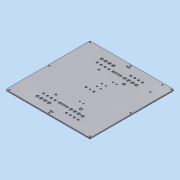
# Autodesk Inventor part: V-Slot Universal Build Pate
Saved by Autodesk Inventor 2013 (Build 170138000, 138)
## iProperties
Created: 2013-12-08
Part Number: V-Slot Universal Build Pate
Material: Aluminum 6061
Document SubType Name: Modeling
Designer: Jon Hollander
Density: 2.71 g/cm^3
Catalog Web Link: www.openbuildspartstore.com
Vendor: OpenBuilds
Mass: 366.388 g
Surface Area: 959.613 cm^2
Volume: 135.198 cm^3
Author: Work
Autodesk Inventor part; units mm, degrees
ref_plane "YZ Plane" through (0, 0, 0) normal (1, 0, 0) x (0, 1, 0)
ref_plane "XZ Plane" through (0, 0, 0) normal (0, 1, 0) x (-1, 0, 0)
ref_plane "XY Plane" through (0, 0, 0) normal (0, 0, 1) x (1, 0, 0)
sketch "Sketch1" plane through (0, 0, 0) normal (0, 0, 1) x (1, 0, 0)
  line L0 (-108, 108) -> (108, 108)
  line L1 (108, 108) -> (108, -108)
  line L2 (108, -108) -> (-108, -108)
  line L3 (-108, -108) -> (-108, 108)
  line L4 (-108, 108) -> (108, -108) construction
  line L5 (108, 108) -> (-108, -108) construction
  point P0 (0, 0)
  dimension "d0" = 216
  dimension "d2" = 216
  constraints: 12 end point, 2 midpoint, 2 parallel, 1 horizontal, 1 perpendicular
  measures "d0" distance of L1.end L2.end
  measures "d2" distance of L2.end L0.start
extrude "Extrusion1" add sketch "Sketch1" along normal mid plane 3
sketch "Sketch2" plane through (0, 0, 1.5) normal (0, 0, 1) x (1, 0, 0)
  line L0 (108, 108) -> (-108, 108) projected
  line L1 (-108, 108) -> (-108, -108) projected
  line L2 (-108, -108) -> (108, -108) projected
  line L3 (108, -108) -> (108, 108) projected
  circle A0 centre (104.5, -104.5) radius 1.8 construction
  line L4 (102.7, -104.5) -> (-104.5, -104.5) construction
  line L5 (104.5, 104.5) -> (-104.5, 104.5) construction
  line L6 (104.5, 104.5) -> (104.5, -104.5) construction
  line L7 (-104.5, 104.5) -> (-104.5, -104.5) construction
  line L8 (0, 104.5) -> (0, -104.5) construction
  point P0 (0, 0)
  point P1 (-102.3056, -104.5)
  point P2 (104.5, 0)
  point P3 (-104.5, 0)
  point P4 (0, 0)
  dimension "d6" = 3.6
  dimension "d5" = 3.5
  dimension "d7" = 1.7
  dimension "d8" = 3.5
  dimension "d9" = 3.5
  dimension "d10" = 3.5
  dimension "d11" = 3.5
  dimension "d13" = 108
  constraints: 10 end point, 3 coincident, 3 midpoint, 3 perpendicular, 2 point on line, 1 horizontal alignment, 1 parallel, 2 other
  measures "d5" distance from line of L3 point (104.5, -104.5)
  measures "d8" distance between parallel lines of L2 L4
  measures "d9" distance between parallel lines of L0 L5
  measures "d10" distance from line of L3 point (104.5, 104.5)
  measures "d11" distance between parallel lines of L1 L7
  measures "d13" distance from line of L3 L8.start
hole "Hole1" at (104.5, 104.5, 1.5) at (104.5, -104.5, 1.5) at (-102.3056, -104.5, 1.5) at (-104.5, 104.5, 1.5) at (104.5, 0, 1.5) at (-104.5, 0, 1.5) at (0, 104.5, 1.5) at (0, -104.5, 1.5) at (0, 0, 1.5) direction (0, 0, -1) diameter 3.6 end through all
sketch "Sketch3" plane through (0, 0, 1.5) normal (0, 0, 1) x (1, 0, 0)
  line L0 (108, 108) -> (-108, 108) projected
  line L1 (-108, 108) -> (-108, -108) projected
  line L2 (108, -108) -> (108, 108) projected
  line L3 (-108, 82.65) -> (108, 82.65) construction
  line L4 (-108, 69) -> (108, 69) construction
  point P0 (-52.3, 82.65)
  point P1 (-42.3, 82.65)
  point P2 (-32.3, 82.65)
  point P3 (-22.3, 82.65)
  point P4 (20.32, 69)
  point P5 (30.32, 69)
  point P6 (40.32, 69)
  point P7 (50.32, 69)
  dimension "d21" = 25.35
  dimension "d23" = 39
  dimension "d24" = 160.3
  dimension "d25" = 150.3
  dimension "d26" = 140.3
  dimension "d27" = 130.3
  dimension "d28" = 57.68
  dimension "d29" = 67.68
  dimension "d30" = 77.68
  dimension "d31" = 87.68
  constraints: 12 point on line, 4 end point, 2 perpendicular
  measures "d21" distance between parallel lines of L0 L3
  measures "d23" distance between parallel lines of L0 L4
  measures "d24" distance from line of L2 point (-52.3, 82.65)
  measures "d25" horizontal distance of L4.end point (-42.3, 82.65)
  measures "d26" distance from line of L2 point (-32.3, 82.65)
  measures "d27" distance from line of L2 point (-22.3, 82.65)
  measures "d28" distance from line of L2 point (50.32, 69)
  measures "d29" distance from line of L2 point (40.32, 69)
  measures "d30" distance from line of L2 point (30.32, 69)
  measures "d31" distance from line of L2 point (20.32, 69)
hole "Hole2" at (-52.3, 82.65, 1.5) at (-42.3, 82.65, 1.5) at (-32.3, 82.65, 1.5) at (-22.3, 82.65, 1.5) at (20.32, 69, 1.5) at (30.32, 69, 1.5) at (40.32, 69, 1.5) at (50.32, 69, 1.5) direction (0, 0, -1) diameter 7.14 end through all
sketch "Sketch4" plane through (0, 0, 1.5) normal (0, 0, 1) x (1, 0, 0)
  line L0 (-108, 108) -> (-108, -108) projected
  line L1 (108, -108) -> (108, 108) projected
  line L2 (-108, 82.65) -> (108, 82.65) construction
  line L3 (-108, 69) -> (108, 69) construction
  point P0 (-50.32, 69)
  point P1 (-40.32, 69)
  point P2 (-30.32, 69)
  point P3 (-20.32, 69)
  point P4 (22.3, 82.65)
  point P5 (32.3, 82.65)
  point P6 (42.3, 82.65)
  point P7 (52.3, 82.65)
  dimension "d125" = 158.32
  dimension "d126" = 148.32
  dimension "d127" = 138.32
  dimension "d128" = 128.32
  dimension "d129" = 55.7
  dimension "d130" = 65.7
  dimension "d131" = 75.7
  dimension "d132" = 85.7
  constraints: 12 point on line, 4 end point, 2 perpendicular
  measures "d125" distance from line of L1 point (-50.32, 69)
  measures "d126" distance from line of L1 point (-40.32, 69)
  measures "d127" distance from line of L1 point (-30.32, 69)
  measures "d128" distance from line of L1 point (-20.32, 69)
  measures "d129" distance from line of L1 point (52.3, 82.65)
  measures "d130" distance from line of L1 point (42.3, 82.65)
  measures "d131" distance from line of L1 point (32.3, 82.65)
  measures "d132" distance from line of L1 point (22.3, 82.65)
hole "Hole3" at (-50.32, 69, 1.5) at (-40.32, 69, 1.5) at (-30.32, 69, 1.5) at (-20.32, 69, 1.5) at (22.3, 82.65, 1.5) at (32.3, 82.65, 1.5) at (42.3, 82.65, 1.5) at (52.3, 82.65, 1.5) direction (0, 0, -1) diameter 5 end through all
sketch "Sketch5" plane through (0, 0, 1.5) normal (0, 0, 1) x (1, 0, 0)
  circle A0 centre (0, 0) radius 1.8 projected
  line L0 (-108, 108) -> (-108, -108) projected
  line L1 (108, -108) -> (108, 108) projected
  line L2 (-108, 55.35) -> (108, 55.35) construction
  point P0 (-32.3, 55.35)
  dimension "d46" = 55.35
  dimension "d47" = 75.7
  constraints: 3 point on line, 2 end point, 1 perpendicular
  measures "d46" distance from line of A0.centre L2
  measures "d47" distance from line of L0 point (-32.3, 55.35)
hole "Hole4" at (-32.3, 55.35, 1.5) direction (0, 0, -1) diameter 5 end through all
sketch "Sketch6" plane through (0, 0, 1.5) normal (0, 0, 1) x (1, 0, 0)
  circle A0 centre (-32.3, 55.35) radius 2.5 projected
  point P0 (32.3, 55.35)
  dimension "d55" = 64.6
  constraints: 1 horizontal alignment
  measures "d55" distance of A0.centre point (32.3, 55.35)
hole "Hole5" at (32.3, 55.35, 1.5) direction (0, 0, -1) diameter 7.14 end through all
mirror "Mirror1" about plane through (0, 0, 0) normal (0, 1, 0) of "Hole2", "Hole3", "Hole4", "Hole5"
sketch "Sketch7" plane through (0, 0, 1.5) normal (0, 0, 1) x (1, 0, 0)
  circle A0 centre (0, 0) radius 1.8 projected
  point P0 (-10, 0)
  point P1 (10, 0)
  dimension "d63" = 10
  dimension "d64" = 10
  measures "d63" distance of A0.centre point (-10, 0)
  measures "d64" distance of A0.centre point (10, 0)
hole "Hole6" at (-10, 0, 1.5) at (10, 0, 1.5) direction (0, 0, -1) diameter 5 end through all
sketch "Sketch8" plane through (0, 0, 1.5) normal (0, 0, 1) x (1, 0, 0)
  line L0 (108, 108) -> (-108, 108) projected
  line L1 (-108, 108) -> (-108, -108) projected
  line L2 (108, -108) -> (108, 108) projected
  line L3 (2.5, 15.2915) -> (2.5, 28) construction
  point P0 (12.64, 15.17)
  point P1 (12.64, 28)
  dimension "d72" = 80
  dimension "d73" = 10.14
  dimension "d74" = 12.83
  dimension "d75" = 110.5
  constraints: 2 end point, 2 parallel, 1 coincident, 1 horizontal alignment, 1 vertical alignment
  measures "d72" distance from line of L0 point (12.64, 28)
  measures "d73" distance of L3.end point (12.64, 28)
  measures "d74" distance of point (12.64, 28) point (12.64, 15.17)
  measures "d75" distance from line of L1 point (2.5, 15.291)
hole "Hole7" at (2.5, 15.2915, 1.5) at (12.64, 15.17, 1.5) at (12.64, 28, 1.5) at (2.5, 28, 1.5) direction (0, 0, -1) diameter 3.5 end through all
sketch "Sketch9" plane through (0, 0, 1.5) normal (0, 0, 1) x (1, 0, 0)
  line L0 (108, 108) -> (-108, 108) projected
  line L1 (-108, 108) -> (-108, -108) projected
  point P0 (14, 45)
  point P1 (23.12, 45)
  dimension "d83" = 122
  dimension "d84" = 63
  dimension "d85" = 9.12
  measures "d83" distance from line of L1 point (14, 45)
  measures "d84" distance from line of L0 point (14, 45)
  measures "d85" distance of point (23.12, 45) point (14, 45)
hole "Hole8" at (14, 45, 1.5) at (23.12, 45, 1.5) direction (0, 0, -1) diameter 3.14 end through all
sketch "Sketch10" plane through (0, 0, 1.5) normal (0, 0, 1) x (1, 0, 0)
  circle A0 centre (14, 45) radius 1.57 projected
  line L0 (-108, -108) -> (108, -108) projected
  line L1 (108, -108) -> (108, 108) projected
  line L2 (14, 45) -> (14, -40) construction
  point P0 (23.12, -40)
  dimension "d93" = 68
  dimension "d94" = 9.12
  constraints: 2 end point, 1 coincident, 1 horizontal alignment, 1 parallel
  measures "d93" distance from line of L2.end L0
  measures "d94" distance of point (23.12, -40) point (14, -40)
hole "Hole9" at (14, -40, 1.5) at (23.12, -40, 1.5) direction (0, 0, -1) diameter 3.14 end through all
sketch "Sketch11" plane through (0, 0, 1.5) normal (0, 0, 1) x (1, 0, 0)
  circle A0 centre (0, -104.5) radius 1.8 projected
  line L0 (-108, -108) -> (108, -108) projected
  line L1 (-3.25, -97.12) -> (3.25, -97.12)
  line L2 (3.25, -97.12) -> (3.25, -100.12)
  line L3 (3.25, -100.12) -> (-3.25, -100.12)
  line L4 (-3.25, -100.12) -> (-3.25, -97.12)
  line L5 (-3.25, -97.12) -> (3.25, -100.12) construction
  line L6 (3.25, -97.12) -> (-3.25, -100.12) construction
  arc A1 (-3.25, -97.12) -> (-3.25, -100.12) centre (-3.25, -98.62) ccw
  arc A2 (3.25, -100.12) -> (3.25, -97.12) centre (3.25, -98.62) ccw
  point P0 (0, -98.62)
  dimension "d104" = 9.38
  dimension "d105" = 6.5
  dimension "d106" = 3
  constraints: 12 end point, 4 midpoint, 4 point on circle, 2 centre point, 2 parallel, 1 horizontal, 1 perpendicular, 1 vertical alignment
  measures "d104" distance from line of L0 point (0, -98.62)
  measures "d105" distance of L1.start L1.end
  measures "d106" distance between parallel lines of L3 L1
extrude "Extrusion2" cut sketch "Sketch11" against normal through all contours L1 L2 L3 L4 | L4 A1 | A2 L2
sketch "Sketch12" plane through (0, 0, 1.5) normal (0, 0, 1) x (1, 0, 0)
  circle A0 centre (0, -104.5) radius 1.8 projected
  line L0 (-108, -108) -> (108, -108) projected
  line L1 (-10, -66.5) -> (10, -66.5)
  line L2 (10, -66.5) -> (10, -71.5)
  line L3 (10, -71.5) -> (-10, -71.5)
  line L4 (-10, -71.5) -> (-10, -66.5)
  line L5 (-10, -66.5) -> (10, -71.5) construction
  line L6 (10, -66.5) -> (-10, -71.5) construction
  arc A1 (-10, -66.5) -> (-10, -71.5) centre (-10, -69) ccw
  arc A2 (10, -71.5) -> (10, -66.5) centre (10, -69) ccw
  point P0 (0, -69)
  dimension "d109" = 5
  dimension "d111" = 39
  dimension "d112" = 20
  constraints: 12 end point, 4 midpoint, 4 point on circle, 2 centre point, 2 parallel, 1 horizontal, 1 perpendicular, 1 vertical alignment
  measures "d109" distance of L1.end L2.end
  measures "d111" distance from line of L0 point (0, -69)
  measures "d112" distance of L1.start L1.end
extrude "Extrusion3" cut sketch "Sketch12" against normal through all contours L1 L2 L3 L4 | L4 A1 | A2 L2
mirror "Mirror2" about plane through (0, 0, 0) normal (0, 1, 0) of "Extrusion2", "Extrusion3"
sketch "Sketch13" plane through (0, 0, 1.5) normal (0, 0, 1) x (1, 0, 0)
  circle A0 centre (104.5, 104.5) radius 1.8 projected
  line L0 (108, 108) -> (-108, 108) projected
  point P0 (83, 102.92)
  point P1 (83, 72)
  dimension "d115" = 1.58
  dimension "d116" = 21.5
  dimension "d117" = 36
  constraints: 1 vertical alignment
  measures "d115" vertical distance of A0.centre point (83, 102.92)
  measures "d116" horizontal distance of A0.centre point (83, 102.92)
  measures "d117" distance from line of L0 point (83, 72)
hole "Hole10" at (83, 102.92, 1.5) at (83, 72, 1.5) direction (0, 0, -1) diameter 3.6 end through all
fillet "Fillet1" radius 1.75 4 edges at (-108, -108, 0) (-108, 108, 0) (108, -108, 0) (108, 108, 0)
body "Solid1"
